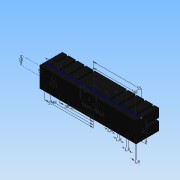
# Autodesk Inventor part: Distance_test_rig
Saved by Autodesk Inventor 2016 (Build 200138000, 138)
## iProperties
Created: 2015-05-18
Part Number: Distance_test_rig
Material: Generic
Document SubType Name: Modeling
Designer: Openlab
Density: 1 g/cm^3
Appearance: Glossy - Black
Author: Openlab
Autodesk Inventor part; units mm, degrees
ref_plane "YZ Plane" through (0, 0, 0) normal (1, 0, 0) x (0, 1, 0)
ref_plane "XZ Plane" through (0, 0, 0) normal (0, 1, 0) x (-1, 0, 0)
ref_plane "XY Plane" through (0, 0, 0) normal (0, 0, 1) x (1, 0, 0)
sketch "Sketch1" plane through (0, 0, 0) normal (0, 1, 0) x (-1, 0, 0)
  line L0 (61.25, -5.25) -> (48.75, -5.25)
  line L1 (48.75, -5.25) -> (48.75, -17.75)
  line L2 (48.75, -17.75) -> (61.25, -17.75)
  line L3 (61.25, -17.75) -> (61.25, -5.25)
  line L4 (110, 0) -> (0, 0)
  line L5 (0, 0) -> (0, -23)
  line L6 (0, -23) -> (110, -23)
  line L7 (110, -23) -> (110, 0)
  line L8 (70.7232, -11.5) -> (42.7232, -11.5) construction
  line L9 (55, -2.25) -> (55, -23.25) construction
  line L10 (37, -23) -> (37, 0)
  line L11 (35.2, 0) -> (35.2, -23)
  line L12 (27, 0) -> (27, -23)
  line L13 (25.2, 0) -> (25.2, -23)
  line L14 (17, 0) -> (17, -23)
  line L15 (15.2, 0) -> (15.2, -23)
  line L16 (7, 0) -> (7, -23)
  line L17 (5.2, -23) -> (5.2, 0)
  line L18 (73, -14.55) -> (71.5, -14.55)
  line L19 (71.5, -14.55) -> (71.5, -8.45)
  line L20 (71.5, -8.45) -> (73, -8.45)
  line L21 (83, -14.55) -> (81.5, -14.55)
  line L22 (81.5, -14.55) -> (81.5, -8.45)
  line L23 (81.5, -8.45) -> (83, -8.45)
  line L24 (93, -14.55) -> (91.5, -14.55)
  line L25 (91.5, -14.55) -> (91.5, -8.45)
  line L26 (91.5, -8.45) -> (93, -8.45)
  line L27 (103, -14.55) -> (101.5, -14.55)
  line L28 (101.5, -14.55) -> (101.5, -8.45)
  line L29 (101.5, -8.45) -> (103, -8.45)
  line L30 (63.25, -13) -> (63.25, -15.5)
  line L31 (63.25, -13) -> (61.25, -13)
  line L32 (61.25, -10) -> (63.25, -10)
  line L33 (48.75, -13) -> (46.75, -13)
  line L34 (46.75, -10) -> (48.75, -10)
  line L35 (103, -17.5) -> (101, -17.5)
  line L36 (101, -17.5) -> (101, -15.5)
  line L37 (101, -15.5) -> (103, -15.5)
  line L38 (103, -7.5) -> (101, -7.5)
  line L39 (101, -7.5) -> (101, -5.5)
  line L40 (101, -5.5) -> (103, -5.5)
  line L41 (137, -16.5) -> (72.25, -16.5) construction
  line L42 (137, -6.5) -> (72.6204, -6.5) construction
  line L43 (104.8, -17.5) -> (106.8, -17.5)
  line L44 (106.8, -17.5) -> (106.8, -15.5)
  line L45 (106.8, -15.5) -> (104.8, -15.5)
  line L46 (104.8, -7.5) -> (106.8, -7.5)
  line L47 (106.8, -7.5) -> (106.8, -5.5)
  line L48 (106.8, -5.5) -> (104.8, -5.5)
  line L49 (104.8, -23) -> (104.8, -17.5)
  line L50 (103, -17.5) -> (103, -23)
  line L51 (104.8, -15.5) -> (104.8, -7.5)
  line L52 (104.8, -5.5) -> (104.8, 0)
  line L53 (103, 0) -> (103, -5.5)
  line L54 (93, -15.5) -> (91, -15.5)
  line L55 (91, -15.5) -> (91, -17.5)
  line L56 (96.8, -17.5) -> (96.8, -15.5)
  line L57 (96.8, -15.5) -> (94.8, -15.5)
  line L58 (94.8, -5.5) -> (96.8, -5.5)
  line L59 (96.8, -5.5) -> (96.8, -7.5)
  line L60 (96.8, -7.5) -> (94.8, -7.5)
  line L61 (91, -7.5) -> (91, -5.5)
  line L62 (91, -7.5) -> (93, -7.5)
  line L63 (91, -5.5) -> (93, -5.5)
  line L64 (91, -17.5) -> (93, -17.5)
  line L65 (94.8, -17.5) -> (96.8, -17.5)
  line L66 (94.8, -17.5) -> (94.8, -23)
  line L67 (93, -17.5) -> (93, -23)
  line L68 (94.8, 0) -> (94.8, -5.5)
  line L69 (94.8, -7.5) -> (94.8, -15.5)
  line L70 (93, 0) -> (93, -5.5)
  line L71 (81, -17.5) -> (81, -15.5)
  line L72 (86.8, -15.5) -> (86.8, -17.5)
  line L73 (86.8, -17.5) -> (84.8, -17.5)
  line L74 (83, -17.5) -> (81, -17.5)
  line L75 (81, -15.5) -> (83, -15.5)
  line L76 (84.8, -15.5) -> (86.8, -15.5)
  line L77 (84.8, -7.5) -> (86.8, -7.5)
  line L78 (86.8, -7.5) -> (86.8, -5.5)
  line L79 (86.8, -5.5) -> (84.8, -5.5)
  line L80 (83, -7.5) -> (81, -7.5)
  line L81 (81, -7.5) -> (81, -5.5)
  line L82 (81, -5.5) -> (83, -5.5)
  line L83 (84.8, -23) -> (84.8, -17.5)
  line L84 (83, -17.5) -> (83, -23)
  line L85 (84.8, -15.5) -> (84.8, -7.5)
  line L86 (84.8, -5.5) -> (84.8, 0)
  line L87 (83, 0) -> (83, -5.5)
  line L88 (73, -15.5) -> (71, -15.5)
  line L89 (71, -15.5) -> (71, -17.5)
  line L90 (71, -17.5) -> (73, -17.5)
  line L91 (74.8, -17.5) -> (76.8, -17.5)
  line L92 (76.8, -17.5) -> (76.8, -15.5)
  line L93 (76.8, -15.5) -> (74.8, -15.5)
  line L94 (74.8, -7.5) -> (76.8, -7.5)
  line L95 (76.8, -7.5) -> (76.8, -5.5)
  line L96 (76.8, -5.5) -> (74.8, -5.5)
  line L97 (73, -5.5) -> (71, -5.5)
  line L98 (71, -5.5) -> (71, -7.5)
  line L99 (73, -7.5) -> (71, -7.5)
  line L100 (74.8, -23) -> (74.8, -17.5)
  line L101 (73, -17.5) -> (73, -23)
  line L102 (74.8, -15.5) -> (74.8, -7.5)
  line L103 (74.8, -5.5) -> (74.8, 0)
  line L104 (73, 0) -> (73, -5.5)
  line L105 (63.25, -15.5) -> (65.05, -15.5)
  line L106 (65.05, -7.5) -> (63.25, -7.5)
  line L107 (63.25, -10) -> (63.25, -7.5)
  line L108 (65.05, -15.5) -> (65.05, -14.1)
  line L109 (65.05, -8.9) -> (65.05, -7.5)
  line L110 (46.75, -7.5) -> (44.95, -7.5)
  line L111 (44.95, -7.5) -> (44.95, -10)
  line L112 (44.95, -13) -> (44.95, -15.5)
  line L113 (44.95, -15.5) -> (46.75, -15.5)
  line L114 (46.75, -15.5) -> (46.75, -13)
  line L115 (67.25, -14.1) -> (67.25, -15.5)
  line L116 (67.25, -15.5) -> (69.05, -15.5)
  line L117 (69.05, -15.5) -> (69.05, -14.1)
  line L118 (69.05, -8.9) -> (69.05, -7.5)
  line L119 (69.05, -7.5) -> (67.25, -7.5)
  line L120 (67.25, -7.5) -> (67.25, -8.9)
  line L121 (42.75, -13) -> (42.75, -15.5)
  line L122 (42.75, -15.5) -> (40.95, -15.5)
  line L123 (40.95, -15.5) -> (40.95, -13)
  line L124 (42.75, -10) -> (42.75, -7.5)
  line L125 (42.75, -7.5) -> (40.95, -7.5)
  line L126 (40.95, -7.5) -> (40.95, -10)
  line L127 (44.95, -13) -> (42.75, -13)
  line L128 (44.95, -10) -> (42.75, -10)
  line L129 (67.25, -14.1) -> (65.05, -14.1)
  line L130 (65.05, -8.9) -> (67.25, -8.9)
  line L131 (103, -7.5) -> (103, -8.45)
  line L132 (103, -14.55) -> (103, -15.5)
  line L133 (104.8, -8.9) -> (110, -8.9)
  line L134 (110, -14.1) -> (104.8, -14.1)
  line L135 (93, -7.5) -> (93, -8.45)
  line L136 (93, -14.55) -> (93, -15.5)
  line L137 (101.5, -14.1) -> (94.8, -14.1)
  line L138 (94.8, -8.9) -> (101.5, -8.9)
  line L139 (91.5, -14.1) -> (84.8, -14.1)
  line L140 (83, -7.5) -> (83, -8.45)
  line L141 (83, -14.55) -> (83, -15.5)
  line L142 (84.8, -8.9) -> (91.5, -8.9)
  line L143 (81.5, -14.1) -> (74.8, -14.1)
  line L144 (71.5, -14.1) -> (69.05, -14.1)
  line L145 (73, -7.5) -> (73, -8.45)
  line L146 (73, -14.55) -> (73, -15.5)
  line L147 (69.05, -8.9) -> (71.5, -8.9)
  line L148 (74.8, -8.9) -> (81.5, -8.9)
  line L149 (40.95, -13) -> (37, -13)
  line L150 (40.95, -10) -> (37, -10)
  line L151 (35.2, -13) -> (27, -13)
  line L152 (35.2, -10) -> (27, -10)
  line L153 (25.2, -13) -> (17, -13)
  line L154 (25.2, -10) -> (17, -10)
  line L155 (15.2, -13) -> (7, -13)
  line L156 (5.2, -13) -> (0, -13)
  line L157 (15.2, -10) -> (7, -10)
  line L158 (5.2, -10) -> (0, -10)
  line L159 (69.05, -14.1) -> (69.05, -8.9)
  line L160 (67.25, -14.1) -> (67.25, -8.9)
  line L161 (65.05, -14.1) -> (65.05, -8.9)
  line L162 (63.25, -13) -> (63.25, -10)
  line L163 (44.95, -13) -> (44.95, -10)
  line L164 (42.75, -13) -> (42.75, -10)
  line L165 (40.95, -13) -> (40.95, -10)
  line L166 (46.75, -7.5) -> (46.75, -10)
  line L167 (46.75, -10) -> (46.75, -13)
  point P0 (55, -11.5)
  dimension "d0" = 12.5
  dimension "d1" = 12.5
  dimension "d3" = 23
  dimension "d18" = 1.8
  dimension "d20" = 1.8
  dimension "d22" = 1.8
  dimension "d24" = 1.8
  dimension "d36" = 6.1
  dimension "d37" = 1.5
  dimension "d62" = 3
  dimension "d94" = 2
  dimension "d95" = 2
  dimension "d96" = 10
  dimension "d97" = 1.8
  dimension "d99" = 1.8
  dimension "d101" = 1.8
  dimension "d103" = 1.8
  dimension "d113" = 8
  dimension "d114" = 1.8
  dimension "d117" = 18
  dimension "d118" = 18
  dimension "d119" = 2
  dimension "d120" = 2
  dimension "d122" = 6
  dimension "d123" = 28
  dimension "d124" = 38
  dimension "d125" = 48
  dimension "d126" = 55
  dimension "d127" = 28
  dimension "d128" = 38
  dimension "d129" = 48
  dimension "d130" = 55
  dimension "d131" = 6
  dimension "d132" = 5.2
  dimension "d133" = 3
  constraints: 333 end point, 129 perpendicular, 86 point on line, 55 collinear, 43 vertical, 23 horizontal, 22 equal length, 11 parallel, 1 coincident, 60 other
  measures "d0" distance of L2.end L1.end
  measures "d1" distance of L0.end L1.end
  measures "d3" distance of L5.end L5.start
  measures "d18" distance between parallel lines of L11 L10
  measures "d20" distance between parallel lines of L13 L12
  measures "d22" distance between parallel lines of L15 L14
  measures "d24" distance between parallel lines of L17 L16
  measures "d36" distance of L27.end L28.end
  measures "d37" distance of L27.start L27.end
  measures "d62" distance between parallel lines of L32 L31
  measures "d94" distance of L35.end L36.end
  measures "d95" distance of L35.start L35.end
  measures "d96" distance between parallel lines of L42 L41
  measures "d97" distance between parallel lines of L53 L52
  measures "d99" distance between parallel lines of L70 L68
  measures "d101" distance between parallel lines of L87 L86
  measures "d103" distance between parallel lines of L104 L103
  measures "d113" distance between parallel lines of L106 L105
  measures "d114" distance between parallel lines of L107 L109
  measures "d117" distance between parallel lines of L9 L101
  measures "d118" distance between parallel lines of L10 L9
  measures "d119" distance between parallel lines of L3 L30
  measures "d120" distance between parallel lines of L114 L1
  measures "d122" distance between parallel lines of L115 L3
  measures "d123" distance between parallel lines of L84 L9
  measures "d124" distance between parallel lines of L67 L9
  measures "d125" distance between parallel lines of L50 L9
  measures "d126" distance between parallel lines of L7 L9
  measures "d127" distance between parallel lines of L12 L9
  measures "d128" distance between parallel lines of L14 L9
  measures "d129" distance between parallel lines of L16 L9
  measures "d130" distance between parallel lines of L5 L9
  measures "d131" distance between parallel lines of L121 L1
  measures "d132" distance between parallel lines of L133 L134
  measures "d133" distance between parallel lines of L158 L156
extrude "Extrusion10" add sketch "Sketch1" against normal blind 6
extrude "Extrusion12" add sketch "Sketch1" along normal blind 5 contours L32 L162 L31 L3 | L1 L33 L167 L34 | L130 L160 L129 L161 | L163 L127 L164 L128 | L147 L19 L144 L159 | L165 L149 L10 L150 | L11 L151 L12 L152 | L13 L153 L14 L154 | L15 L155 L16 L157 | L148 L22 L143 L102 | L17 L156 L5 L158 | L142 L25 L139 L85 | L7 L134 L51 L133 | L138 L28 L137 L69
extrude "Extrusion13" add sketch "Sketch1" along normal blind 20 contours L0 L1 L34 L166 L110 L111 L128 L124 L125 L126 L150 L10 L4 L104 L97 L98 L99 L145 L20 L19 L147 L118 L119 L120 L130 L109 L106 L107 L32 L3 | L31 L30 L105 L108 L129 L115 L116 L117 L144 L19 L18 L146 L88 L89 L90 L101 L6 L10 L149 L123 L122 L121 L127 L112 L113 L114 L33 L1 L2 L3 | L11 L152 L12 L4 | L6 L12 L151 L11 | L4 L87 L82 L81 L80 L140 L23 L22 L148 L102 L94 L95 L96 L103 | L100 L91 L92 L93 L102 L143 L22 L21 L141 L75 L71 L74 L84 L6 | L13 L154 L14 L4 | L6 L14 L153 L13 | L4 L70 L63 L61 L62 L135 L26 L25 L142 L85 L77 L78 L79 L86 | L83 L73 L72 L76 L85 L139 L25 L24 L136 L54 L55 L64 L67 L6 | L15 L157 L16 L4 | L6 L16 L155 L15 | L4 L53 L40 L39 L38 L131 L29 L28 L138 L69 L60 L59 L58 L68 | L66 L65 L56 L57 L69 L137 L28 L27 L132 L37 L36 L35 L50 L6 | L17 L158 L5 L4 | L6 L5 L156 L17 | L4 L7 L133 L51 L46 L47 L48 L52 | L49 L43 L44 L45 L51 L134 L7 L6
body "Solid3"
